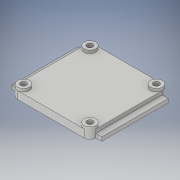
# Autodesk Inventor part: L298N-holder
Saved by Autodesk Inventor 2018 (Build 220112000, 112)
## iProperties
Created: 2018-07-29
Part Number: L298N-holder
Material: Generic
Document SubType Name: Modeling
Designer: jklei
Density: 1 g/cm^3
Appearance: Default
Author: jklei
Autodesk Inventor part; units mm, degrees
ref_plane "YZ Plane" through (0, 0, 0) normal (1, 0, 0) x (0, 1, 0)
ref_plane "XZ Plane" through (0, 0, 0) normal (0, 1, 0) x (-1, 0, 0)
ref_plane "XY Plane" through (0, 0, 0) normal (0, 0, 1) x (1, 0, 0)
sketch "Sketch1" plane through (0, 0, 0) normal (0, 1, 0) x (-1, 0, 0)
  line L0 (0, 0) -> (40.005, 0)
  line L1 (40.005, 0) -> (40.005, -40.0202)
  line L2 (40.005, -40.0202) -> (0, -40.0202)
  line L3 (0, -40.0202) -> (0, 0)
  dimension "d26" = 40.005
  dimension "d27" = 40.0202
  constraints: 8 end point, 2 parallel, 1 horizontal, 1 perpendicular
  measures "d26" distance of L1.end L2.end
  measures "d27" distance of L0.end L1.end
extrude "Extrusion1" add sketch "Sketch1" along normal blind 4
sketch "Sketch2" plane through (0, 4, 0) normal (0, 1, 0) x (1, 0, 0)
  line L0 (-40.0202, 0) -> (0, 0) projected
  line L1 (0, 0) -> (0, 40) projected
  line L2 (0, 40) -> (-40.0202, 40) projected
  line L3 (-40.0202, 40) -> (-40.0202, 0) projected
  line L4 (-37.0202, 37) -> (-3, 37)
  line L5 (-3, 37) -> (-3, 3)
  line L6 (-3, 3) -> (-37.0202, 3)
  line L7 (-37.0202, 3) -> (-37.0202, 37)
  circle A0 centre (-37.0202, 37) radius 1.5
  circle A1 centre (-3, 37) radius 1.5
  circle A2 centre (-3, 3) radius 1.5
  circle A3 centre (-37.0202, 3) radius 1.5
  dimension "d4" = 3
  dimension "d5" = 3
  dimension "d6" = 3
  dimension "d7" = 3
  dimension "d8" = 3
  constraints: 8 end point, 4 centre point, 4 coincident, 3 other
  measures "d4" distance between parallel lines of L2 L4
  measures "d5" diameter of A0
  measures "d6" diameter of A1
  measures "d7" diameter of A2
  measures "d8" diameter of A3
extrude "Extrusion2" cut sketch "Sketch2" against normal blind 4 contours L7 A0 L4 | L4 A0 L7 | A1 L5 L4 | L4 L5 A1 | A3 L6 L7 | L7 L6 A3 | A2 L6 L5 | L5 L6 A2
sketch "Sketch3" plane through (0, 4, 0) normal (0, 1, 0) x (1, 0, 0)
  circle A0 centre (-37.0202, 3) radius 1.5 projected
  circle A1 centre (-37.0202, 37) radius 1.5 projected
  circle A2 centre (-3, 37) radius 1.5 projected
  circle A3 centre (-3, 3) radius 1.5 projected
  circle A4 centre (-37.0202, 3) radius 1.5 projected
  circle A5 centre (-3, 37) radius 1.5 projected
  circle A6 centre (-37.0202, 37) radius 1.5 projected
  circle A7 centre (-3, 3) radius 1.5 projected
  line L0 (-40.005, 0) -> (0, 0) projected
  line L1 (0, 0) -> (0, 40.0202) projected
  line L2 (0, 40.0202) -> (-40.005, 40.0202) projected
  line L3 (-40.005, 40.0202) -> (-40.005, 0) projected
  circle A8 centre (-3, 37) radius 3
  circle A9 centre (-3, 3) radius 3
  circle A10 centre (-37.0202, 3) radius 3
  circle A11 centre (-37.0202, 37) radius 2.9848
  constraints: 4 centre point, 4 coincident, 4 tangent
extrude "Extrusion3" add sketch "Sketch3" along normal blind 1.5 contours A8 | A11 | A10 L3 | A10 L3 | A9
sketch "Sketch4" plane through (0, 0, 0) normal (0, -1, 0) x (1, 0, 0)
  circle A0 centre (-3, -37) radius 1.5 projected
  circle A1 centre (-37.0202, -37) radius 1.5 projected
  circle A2 centre (-37.0202, -3) radius 1.5 projected
  circle A3 centre (-3, -3) radius 1.5 projected
  circle A4 centre (-3, -3) radius 2.5
  circle A5 centre (-3, -37) radius 2.5
  circle A6 centre (-37.0202, -37) radius 2.5
  circle A7 centre (-37.0202, -3) radius 2.5
  point P0 (0, 0)
  dimension "d14" = 5
  dimension "d15" = 5
  dimension "d16" = 5
  dimension "d17" = 5
  constraints: 4 centre point, 4 coincident
  measures "d14" diameter of A4
  measures "d15" diameter of A5
  measures "d16" diameter of A6
  measures "d17" diameter of A7
extrude "Extrusion4" cut sketch "Sketch4" against normal blind 3
fillet "Fillet2" radius 3 4 edges at (-40.005, 2, -40.0202) (-40.005, 2, 0) (0, 2, 0) (0, 2, -40.0202)
sketch "Sketch7" plane through (0, 0, -3) normal (1, 0, 0) x (0, 0, -1)
  line L0 (34.0202, 4) -> (34.0202, 0) projected
  line L1 (0, 0) -> (34.0202, 0)
  line L2 (34.0202, 0) -> (34.0202, 2)
  line L3 (34.0202, 2) -> (0, 2)
  line L4 (0, 2) -> (0, 0)
  point P0 (-3, 0)
  dimension "d29" = 2
  constraints: 8 end point, 2 parallel, 1 horizontal, 1 midpoint, 1 perpendicular
  measures "d29" distance of L2.end L1.end
extrude "Extrusion7" add sketch "Sketch7" along normal blind 3
sketch "Sketch8" plane through (-40.005, 4, -37) normal (-1, 0, 0) x (0, 0, 1)
  line L0 (34, -4) -> (-0.0202, -4) projected
  line L1 (-0.0202, -4) -> (-0.0202, -2) projected
  line L2 (-0.0202, -2) -> (34, -2) projected
  line L3 (34, -2) -> (34, -4) projected
  point P0 (37, -4)
extrude "Extrusion8" add sketch "Sketch8" along normal blind 3
body "Solid1"
